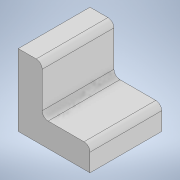
# Autodesk Inventor part: Practice 6
Saved by Autodesk Inventor 2020 (Build 240168000, 168)
## iProperties
Created: 2020-01-23
Part Number: Practice 6
Material: Generic
Document SubType Name: Modeling
Designer: cks4a449
Density: 1 g/cm^3
Appearance: Default
Author: cks4a449
Autodesk Inventor part; units mm, degrees
ref_plane "YZ Plane" through (0, 0, 0) normal (1, 0, 0) x (0, 1, 0)
ref_plane "XZ Plane" through (0, 0, 0) normal (0, 1, 0) x (-1, 0, 0)
ref_plane "XY Plane" through (0, 0, 0) normal (0, 0, 1) x (1, 0, 0)
sketch "Sketch1" plane through (0, 0, 0) normal (0, 0, 1) x (1, 0, 0)
  line L0 (0, 0) -> (0, 38.1)
  line L1 (0, 38.1) -> (12.7, 38.1)
  line L2 (12.7, 38.1) -> (12.7, 12.7)
  line L3 (12.7, 12.7) -> (38.1, 12.7)
  line L4 (38.1, 12.7) -> (38.1, 0)
  line L5 (38.1, 0) -> (0, 0)
  dimension "d0" = 38.1
  dimension "d1" = 12.7
  dimension "d2" = 25.4
  dimension "d3" = 25.4
  dimension "d4" = 12.7
  constraints: 12 end point, 4 perpendicular, 1 vertical
  measures "d0" distance of L0.start L0.end
  measures "d1" distance of L0.end L1.end
  measures "d2" distance of L1.end L2.end
  measures "d3" distance of L2.end L3.end
  measures "d4" distance of L3.end L4.end
extrude "Extrusion1" add sketch "Sketch1" along normal blind 38.1
fillet "Fillet1" radius 3.175 3 edges at (12.7, 38.1, 19.05) (12.7, 12.7, 19.05) (38.1, 12.7, 19.05)
body "Solid1"
